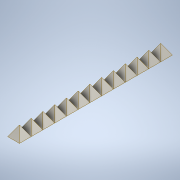
# Autodesk Inventor part: pyr
Saved by Autodesk Inventor 2020 (Build 240168000, 168)
## iProperties
Created: 2020-05-01
Part Number: pyr
Material: Titanium
Document SubType Name: Modeling
Designer: marah
Density: 4.51 g/cm^3
Appearance: Titanium
Mass: 0.456976 g
Surface Area: 3.51 cm^2
Volume: 0.101325 cm^3
Author: marah
Autodesk Inventor part; units mm, degrees
ref_plane "YZ Plane" through (0, 0, 0) normal (1, 0, 0) x (0, 1, 0)
ref_plane "XZ Plane" through (0, 0, 0) normal (0, 1, 0) x (-1, 0, 0)
ref_plane "XY Plane" through (0, 0, 0) normal (0, 0, 1) x (1, 0, 0)
sketch "Sketch1" plane through (0, 0, 0) normal (0, 1, 0) x (-1, 0, 0)
  line L0 (-2.033, 0.9835) -> (0.967, 0.9835)
  line L1 (0.967, 0.9835) -> (0.967, -2.0165)
  line L2 (0.967, -2.0165) -> (-2.033, -2.0165)
  line L3 (-2.033, -2.0165) -> (-2.033, 0.9835)
  point P0 (0, 0)
  dimension "d0" = 3
  dimension "d1" = 3
  constraints: 8 end point, 2 parallel, 1 horizontal, 1 perpendicular
  measures "d0" distance of L0.start L0.end
  measures "d1" distance of L0.end L1.end
extrude "Extrusion1" add sketch "Sketch1" along normal blind 3 draft -30
pattern_linear "Rectangular Pattern1" count 13 spacing 3 along (0, 0, 1) of "Extrusion1" first direction both ways yes
body "Solid1"
